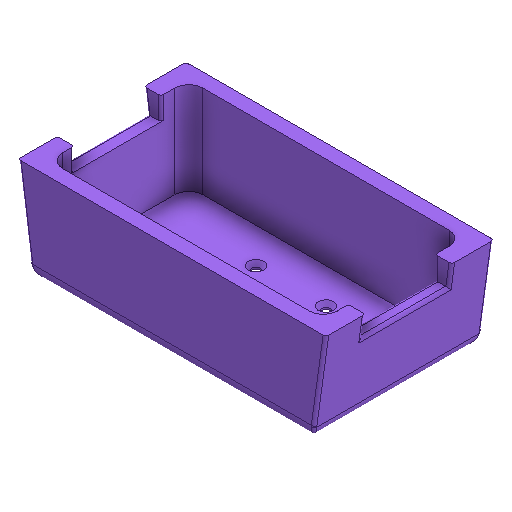
# Autodesk Inventor part: лоток для маркеров
Saved by Autodesk Inventor 2025 (Build 290162000, 162)
## iProperties
Created: 2025-03-03
Part Number: лоток для маркеров
Material: Полиэтилен, высокая плотность
Document SubType Name: Modeling
Designer: volko
Density: 0.952 g/cm^3
Appearance: Фиолетовый
Mass: 421.318 g
Surface Area: 1281.5 cm^2
Volume: 442.561 cm^3
Author: volko
Autodesk Inventor part; units mm, degrees
ref_plane "YZ Plane" through (0, 0, 0) normal (1, 0, 0) x (0, 1, 0)
ref_plane "XZ Plane" through (0, 0, 0) normal (0, 1, 0) x (-1, 0, 0)
ref_plane "XY Plane" through (0, 0, 0) normal (0, 0, 1) x (1, 0, 0)
sketch "Эскиз1" plane through (0, 0, 0) normal (0, 1, 0) x (-1, 0, 0)
  line L0 (98, 50) -> (-98, 50)
  line L1 (-98, 50) -> (-98, -50)
  line L2 (-98, -50) -> (98, -50)
  line L3 (98, -50) -> (98, 50)
  line L4 (110, 60) -> (-110, 60)
  line L5 (-110, 60) -> (-110, -60)
  line L6 (-110, -60) -> (110, -60)
  line L7 (110, -60) -> (110, 60)
  line L8 (154, 0) -> (-154, 0) projected
  line L9 (0, -84) -> (0, 84) projected
  point P0 (0, 0)
  point P1 (0, -60)
  point P2 (0, -50)
  point P3 (0, 50)
  point P4 (0, 60)
  dimension "d1" = 220
  dimension "d2" = 12
  dimension "d3" = 10
  dimension "d4" = 120
  constraints: 16 end point, 4 parallel, 2 horizontal, 2 perpendicular, 4 other
  measures "d1" distance of L4.start L4.end
  measures "d2" distance between parallel lines of L7 L3
  measures "d3" distance between parallel lines of L4 L0
  measures "d4" distance of L4.end L5.end
extrude "Выдавливание1" add sketch "Эскиз1" along normal blind 70 contours L0 L9 L4 L7 L8 L3 | L0 L1 L8 L5 L4 L9 | L8 L7 L6 L9 L2 L3 | L1 L2 L9 L6 L5 L8
extrude "Выдавливание2" add sketch "Эскиз1" along normal blind 4
draft "НаклГрань1" angle 8 pull direction (0, -1, 0) faces at (110, 23.3333, 20) (-110, 23.3333, -20) fixed edges at (110, 70, 0) (-110, 70, 0)
sketch "Эскиз4" plane through (0, 0, 0) normal (1, 0, 0) x (0, 1, 0)
  line L0 (70, -50) -> (70, 50) projected
  line L1 (70, 32) -> (54, 32)
  line L2 (54, 32) -> (54, -30)
  line L3 (54, -30) -> (70, -30)
  line L4 (70, 32) -> (70, -30)
  point P0 (0, 0)
  constraints: 8 end point, 2 perpendicular, 2 point on line, 1 collinear, 1 horizontal
extrude "Выдавливание3" cut sketch "Эскиз4" along normal through all both and the other way through all
fillet "Сопряжение1" radius 10 8 edges at (-98, 37, 50) (-98, 37, -50) (98, 37, -50) (98, 37, 50) (0, 0, 60) (0, 0, -60) (100.1621, 0, 0) (-100.1621, 0, 0)
fillet "Сопряжение2" radius 2 23 edges at (98, 62, -30) (98, 62, 32) (98, 54, 1) (107.7513, 54, 1) (108.8757, 62, 32) (108.8757, 62, -30) (-108.8757, 62, -30) (-107.7513, 54, 1) (-98, 62, -30) (-108.8757, 62, 32) (-98, 62, 32) (-101.4695, 9.3024, 59.9756) (-98.0299, 2.4529, 56.5606) (-105.7838, 40, 60) (-101.4695, 9.3024, -59.9756) (-98.0299, 2.4529, -56.5606) (-105.7838, 40, -60) (101.4695, 9.3024, -59.9756) (98.0299, 2.4529, -56.5606) (105.7838, 40, -60) (101.4695, 9.3024, 59.9756) (98.0299, 2.4529, 56.5606) (105.7838, 40, 60)
sketch "Эскиз5" plane through (0, 4, 0) normal (0, 1, 0) x (1, 0, 0)
  line L0 (0, 84) -> (0, -84) projected
  line L1 (-154, 0) -> (154, 0) projected
  point P0 (0, 0)
  point P1 (-25, 25)
  point P2 (25, 25)
  point P3 (25, -25)
  point P4 (-25, -25)
  dimension "d31" = 25
  dimension "d32" = 25
  constraints: 4 symmetric about line
  measures "d31" distance from line of L1 point (-25, 25)
  measures "d32" distance from line of point (25, 25) L0
hole "Отверстие1" at (-25, 4, -25) at (25, 4, -25) at (25, 4, 25) at (-25, 4, 25) direction (0, -1, 0) diameter 5.5 end through all countersink diameter 11 countersink angle 90
sketch "Эскиз6" plane through (0, 4, 0) normal (0, 1, 0) x (1, 0, 0)
  line L0 (-154, 0) -> (154, 0) projected
  line L1 (0, 84.0012) -> (0, -84.0012) projected
  point P0 (0, 0)
